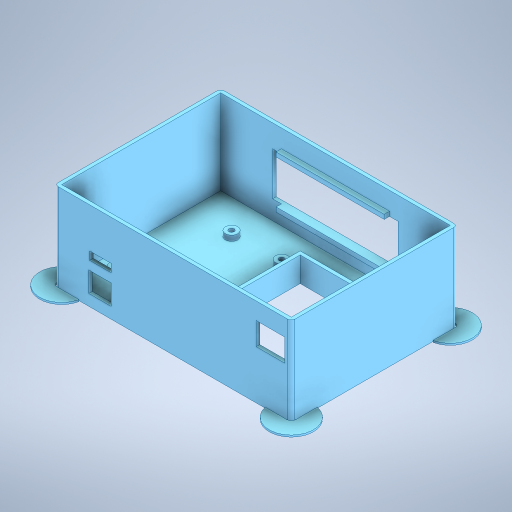
# Autodesk Inventor part: case_under_v2
Saved by Autodesk Inventor 2023 (Build 270158000, 158)
## iProperties
Created: 2022-09-15
Part Number: case_under_v2
Material: 일반
Document SubType Name: Modeling
Designer: 전상현
Density: 1 g/cm^3
Appearance: 기본값(1)
Author: 전상현
Autodesk Inventor part; units mm, degrees
ref_plane "YZ Plane" through (0, 0, 0) normal (1, 0, 0) x (0, 1, 0)
ref_plane "XZ Plane" through (0, 0, 0) normal (0, 1, 0) x (-1, 0, 0)
ref_plane "XY Plane" through (0, 0, 0) normal (0, 0, 1) x (1, 0, 0)
sketch "스케치1" plane through (0, 0, 0) normal (0, 1, 0) x (-1, 0, 0)
  line L0 (65, -45) -> (-65, -45)
  line L1 (-65, -45) -> (-65, 45)
  line L2 (-65, 45) -> (65, 45)
  line L3 (65, 45) -> (65, -45)
  line L4 (65, -45) -> (-65, 45) construction
  line L5 (-65, -45) -> (65, 45) construction
  line L6 (-67, -47) -> (67, -47)
  line L7 (67, -47) -> (67, 47)
  line L8 (67, 47) -> (-67, 47)
  line L9 (-67, 47) -> (-67, -47)
  line L10 (-1, -24) -> (-64, -24)
  line L11 (-64, -24) -> (-64, 34)
  line L12 (-64, 34) -> (-1, 34)
  line L13 (-1, 34) -> (-1, -24)
  circle A0 centre (-32.5, 39) radius 1.5
  circle A1 centre (-32.5, 39) radius 3.5
  arc A2 (-27.5, 39) -> (-37.5, 39) centre (-32.5, 39) ccw
  line L14 (-27.5, 39) -> (-27.5, 34)
  line L15 (-37.5, 39) -> (-37.5, 34)
  point P0 (0, 0)
  point P1 (-32.5, 34)
  point P2 (-32.5, 44)
  dimension "d0" = 130
  dimension "d1" = 90
  dimension "d2" = 2
  dimension "d3" = 58
  dimension "d4" = 63
  dimension "d5" = 3
  dimension "d6" = 7
  dimension "d7" = 10
  dimension "d8" = 1
  dimension "d9" = 1
  constraints: 32 end point, 6 parallel, 5 perpendicular, 4 midpoint, 3 centre point, 3 point on circle, 2 coincident, 2 horizontal, 2 point on line, 2 tangent, 2 vertical alignment, 3 other
  measures "d0" distance of L1.end L2.end
  measures "d1" distance of L0.end L1.end
  measures "d2" distance between parallel lines of L0 L6
  measures "d3" distance of L10.end L11.end
  measures "d4" distance of L10.start L10.end
  measures "d5" diameter of A0
  measures "d6" diameter of A1
  measures "d7" diameter of A2
  measures "d8" distance from line of L2 point (-32.5, 44)
  measures "d9" distance between parallel lines of L1 L11
extrude "돌출1" add sketch "스케치1" along normal blind 2 contours L0 L1 L2 L3 | L9 L8 L7 L6
extrude "돌출2" add sketch "스케치1" along normal blind 3 from surface at 2 contours L12 L15 A2 L14 | A1
sketch "스케치2" plane through (0, 2, 0) normal (0, 1, 0) x (1, 0, 0)
  line L0 (-67, -47) -> (67, -47) projected
  line L1 (67, -47) -> (67, 47) projected
  line L2 (67, 47) -> (-67, 47) projected
  line L3 (-67, 47) -> (-67, -47) projected
  line L4 (64, -34) -> (37.5, -34) projected
  line L5 (37.5, -34) -> (37.5, -39) projected
  arc A0 (27.5, -39) -> (37.5, -39) centre (32.5, -39) ccw projected
  line L6 (27.5, -39) -> (27.5, -34) projected
  line L7 (27.5, -34) -> (1, -34) projected
  line L8 (1, -34) -> (1, 24) projected
  line L9 (1, 24) -> (64, 24) projected
  line L10 (64, 24) -> (64, -34) projected
  line L11 (39, -39) -> (39, -35.5)
  line L12 (64, -55.5) -> (65.5, -55.5)
  line L13 (65.5, -55.5) -> (65.5, 25.5)
  line L14 (65.5, 25.5) -> (-0.5, 25.5)
  line L15 (-0.5, 25.5) -> (-0.5, -55.5)
  line L16 (-0.5, -55.5) -> (1, -55.5)
  line L17 (26, -55.5) -> (26, -39)
  arc A1 (26, -39) -> (39, -39) centre (32.5, -39) ccw
  line L18 (39, -35.5) -> (39, -34)
  line L19 (26, -55.5) -> (26, -34)
  point P0 (0, 0)
  dimension "d14" = 1.5
  constraints: 18 end point, 4 point on line, 2 point on circle, 1 centre point, 1 collinear, 1 parallel, 1 tangent, 1 vertical, 3 other
  measures "d14" radial gap between concentric circles of A0 A1
extrude "돌출3" add sketch "스케치2" along normal blind 3 contours L19 L7 L6 A0 L5 L4 L18 L11 A1
fillet "모깎기1" radius 1 2 edges at (32.5, 2, 45.5) (39, 2, 36.5)
extrude "돌출4" add sketch "스케치1" along normal blind 50 contours L9 L8 L7 L6
sketch "스케치3" plane through (0, 2, 0) normal (0, 1, 0) x (1, 0, 0)
  point P0 (0, 0)
sketch "스케치4" plane through (0, 2, 0) normal (0, 1, 0) x (1, 0, 0)
  line L0 (37, -45) -> (65, -45) projected
  line L1 (65, -45) -> (65, 45) projected
  line L2 (65, 45) -> (-65, 45) projected
  line L3 (-65, 45) -> (-65, -45) projected
  line L4 (-65, -45) -> (28, -45) projected
  arc A0 (25, -39) -> (28, -45) centre (32.5, -39) ccw projected
  line L5 (25, -34) -> (1, -34) projected
  line L6 (1, -34) -> (1, 24) projected
  line L7 (1, 24) -> (64, 24) projected
  line L8 (64, 24) -> (64, -34) projected
  line L9 (64, -34) -> (40, -34) projected
  line L10 (40, -39) -> (40, -34) projected
  arc A1 (37, -45) -> (40, -39) centre (32.5, -39) ccw projected
  line L11 (73.9957, 33.9957) -> (-8.9957, 33.9957)
  line L12 (-8.9957, 33.9957) -> (-8.9957, -43.9957)
  line L13 (-8.9957, -43.9957) -> (25.1098, -43.9957)
  line L14 (49.9957, -39) -> (49.9957, -43.9957)
  line L15 (49.9957, -43.9957) -> (73.9957, -43.9957)
  line L16 (73.9957, -43.9957) -> (73.9957, 33.9957)
  line L17 (-1, 26) -> (74.9957, 26)
  line L18 (74.9957, 26) -> (74.9957, -36)
  line L19 (74.9957, -36) -> (-1, -36)
  line L20 (-1, -36) -> (-1, 26)
  line L21 (25.1098, -36) -> (49.9957, -36)
  line L22 (49.9957, -43.9957) -> (25.1098, -43.9957)
  line L23 (25, -34) -> (25, -39) projected
  line L24 (25, -34) -> (40, -34)
  line L25 (64, -34) -> (37.5, -34) projected
  line L26 (25.1098, -36) -> (40, -36)
  point P0 (0, 0)
  point P1 (40, -36)
  point P2 (25, -36)
  point P3 (73.9957, -36)
  point P4 (73.9957, 26)
  point P5 (65, -36)
  point P6 (65, 26)
  dimension "d20" = 2
  dimension "d21" = 2
  dimension "d22" = 2
  dimension "d23" = 1
  constraints: 28 end point, 5 point on line, 3 parallel, 2 horizontal, 1 collinear, 1 perpendicular, 4 other
  measures "d20" distance between parallel lines of L17 L7
  measures "d21" distance between parallel lines of L9 L19
  measures "d22" distance between parallel lines of L6 L20
  measures "d23" distance between parallel lines of L18 L16
extrude "돌출5" add sketch "스케치4" along normal blind 12 contours L19 L10 L9 L8 L7 L6 L5 L23 L20 L17 L1 | L19 L23 L24 L10
sketch "스케치5" plane through (74.9957, 2, -26) normal (0, 0, -1) x (-1, 0, 0)
  line L0 (37.4957, 2.5) -> (47.4957, 2.5)
  line L1 (47.4957, 2.5) -> (47.4957, 0)
  line L2 (47.4957, 0) -> (37.4957, 0)
  line L3 (37.4957, 0) -> (37.4957, 2.5)
  line L4 (9.9957, 0) -> (75.9957, 0) projected
  line L5 (0, 0) -> (0, 12) projected
  point P0 (74.9957, -2)
  point P1 (39.9957, 0)
  point P2 (42.4957, 2.5)
  point P3 (10.9957, 12)
  point P4 (7.9957, 0)
  dimension "d28" = 2.5
  dimension "d29" = 10
  dimension "d93" = 31.5
  constraints: 8 end point, 2 parallel, 1 horizontal, 1 midpoint, 1 perpendicular, 1 point on line
  measures "d28" distance of L0.end L1.end
  measures "d29" distance of L0.start L0.end
  measures "d93" horizontal distance of point (10.996, 12) point (42.496, 2.5)
extrude "돌출6" cut sketch "스케치5" against normal up to surface (2 mm away)
sketch "스케치6" plane through (0, 2, 0) normal (0, 1, 0) x (1, 0, 0)
  line L0 (-3.7, -40.4) -> (-57, -40.4)
  line L1 (-57, -40.4) -> (-57, 28.2)
  line L2 (-57, 28.2) -> (-3.7, 28.2)
  line L3 (-3.7, 28.2) -> (-3.7, -40.4)
  line L4 (-3.7, 25.7) -> (-51.0807, 25.7)
  line L5 (-51.0807, 25.7) -> (-51.0807, 28.2)
  line L6 (-51.0807, 28.2) -> (-3.7, 28.2)
  line L7 (-3.7, 28.2) -> (-3.7, 25.7)
  line L8 (-51.0807, 25.7) -> (-57, 25.7)
  circle A0 centre (-11.15, 25.7) radius 1.5
  circle A1 centre (-39.55, 25.7) radius 1.5
  circle A2 centre (-54.75, -24.8) radius 1.5
  circle A3 centre (-6.45, -26.7) radius 1.5
  line L9 (-35.4, -40.4) -> (-47.4, -40.4)
  line L10 (-47.4, -40.4) -> (-47.4, -47)
  line L11 (-47.4, -47) -> (-35.4, -47)
  line L12 (-35.4, -47) -> (-35.4, -40.4)
  line L13 (-67, -47) -> (67, -47) projected
  line L14 (-65, -45) -> (-65, 45) projected
  circle A4 centre (-54.75, -24.8) radius 3.5
  circle A5 centre (-6.45, -26.7) radius 3.5
  circle A6 centre (-11.15, 25.7) radius 3.5
  circle A7 centre (-39.55, 25.7) radius 3.5
  point P0 (0, 0)
  point P1 (-41.4, -47)
  point P2 (-54.0404, 25.7)
  dimension "d33" = 53.3
  dimension "d34" = 68.6
  dimension "d36" = 3
  dimension "d37" = 3
  dimension "d38" = 28.4
  dimension "d39" = 3
  dimension "d40" = 3
  dimension "d41" = 52.4
  dimension "d42" = 50.5
  dimension "d44" = 15.2
  dimension "d45" = 4.7
  dimension "d46" = 2.25
  dimension "d47" = 12
  dimension "d48" = 9.6
  dimension "d49" = 6.6
  dimension "d50" = 8
  dimension "d51" = 2.5
  dimension "d52" = 2
  dimension "d53" = 2
  dimension "d54" = 2
  dimension "d55" = 2
  constraints: 26 end point, 8 centre point, 7 point on line, 6 parallel, 4 horizontal, 3 perpendicular, 2 midpoint
  measures "d33" distance of L0.start L0.end
  measures "d34" distance of L0.end L1.end
  measures "d36" diameter of A0
  measures "d37" diameter of A1
  measures "d38" distance of A1.centre A0.centre
  measures "d39" diameter of A2
  measures "d40" diameter of A3
  measures "d41" distance from line of L4 A3.centre
  measures "d42" distance from line of L8 A2.centre
  measures "d44" horizontal distance of A1.centre A2.centre
  measures "d45" horizontal distance of A0.centre A3.centre
  measures "d46" distance from line of L1 A2.centre
  measures "d47" distance of L10.end L11.end
  measures "d48" distance between parallel lines of L1 L10
  measures "d49" distance of L9.end L10.end
  measures "d50" distance between parallel lines of L14 L1
  measures "d51" distance from line of L2 point (-54.04, 25.7)
  measures "d52" radial gap between concentric circles of A2 A4
  measures "d53" radial gap between concentric circles of A3 A5
  measures "d54" radial gap between concentric circles of A0 A6
  measures "d55" radial gap between concentric circles of A1 A7
extrude "돌출7" add sketch "스케치6" along normal blind 3 contours A5 L3 | L3 A5 | A4 L1 | L1 A4 | A6 L4 A0 | L4 A0 A6 L2 | L2 A6 | A7 L4 A1 | L4 A1 A7 L2 | L2 A7
sketch "스케치7" plane through (65, 50, 45) normal (0, 0, -1) x (-1, 0, 0)
  line L0 (100.4, -32.5) -> (112.4, -32.5)
  line L1 (112.4, -32.5) -> (112.4, -43.4)
  line L2 (112.4, -43.4) -> (100.4, -43.4)
  line L3 (100.4, -43.4) -> (100.4, -32.5)
  line L4 (130, -48) -> (130, 0) projected
  line L5 (130, -48) -> (37, -48) projected
  line L6 (112.7, -32.2) -> (100.1, -32.2)
  line L7 (100.1, -32.2) -> (100.1, -43.7)
  line L8 (100.1, -43.7) -> (112.7, -43.7)
  line L9 (112.7, -43.7) -> (112.7, -32.2)
  point P0 (65, -50)
  dimension "d58" = 10.9
  dimension "d59" = 12
  dimension "d60" = 17.6
  dimension "d61" = 4.6
  dimension "d62" = 0.3
  constraints: 16 end point, 4 parallel, 2 perpendicular, 1 horizontal, 3 other
  measures "d58" distance of L0.end L1.end
  measures "d59" distance of L0.start L0.end
  measures "d60" distance between parallel lines of L4 L1
  measures "d61" distance between parallel lines of L5 L2
  measures "d62" distance between parallel lines of L0 L6
extrude "돌출8" cut sketch "스케치7" against normal through all contours L0 L1 L2 L3 | L9 L8 L7 L6
sketch "스케치8" plane through (67, 0, -47) normal (0, 0, -1) x (-1, 0, 0)
  line L0 (31.4, 37.25) -> (102.6, 37.25)
  line L1 (102.6, 37.25) -> (102.6, 12.75)
  line L2 (102.6, 12.75) -> (31.4, 12.75)
  line L3 (31.4, 12.75) -> (31.4, 37.25)
  line L4 (31.4, 37.25) -> (102.6, 12.75) construction
  line L5 (102.6, 37.25) -> (31.4, 12.75) construction
  line L6 (27, 43) -> (107, 43)
  line L7 (107, 43) -> (107, 7)
  line L8 (107, 7) -> (27, 7)
  line L9 (27, 7) -> (27, 43)
  line L10 (27, 43) -> (107, 7) construction
  line L11 (107, 43) -> (27, 7) construction
  circle A0 centre (104.5, 40.5) radius 1.6
  circle A1 centre (104.5, 9.5) radius 1.6
  circle A2 centre (29.5, 9.5) radius 1.6
  circle A3 centre (29.5, 40.5) radius 1.6
  line L12 (134, 0) -> (134, 50) projected
  point P0 (67, 0)
  point P1 (67, 25)
  point P2 (134, 25)
  dimension "d65" = 71.2
  dimension "d66" = 24.5
  dimension "d67" = 36
  dimension "d68" = 80
  dimension "d69" = 3.2
  dimension "d70" = 2.5
  dimension "d71" = 3.2
  dimension "d72" = 3.2
  dimension "d73" = 3.2
  dimension "d74" = 2.5
  dimension "d75" = 31
  dimension "d76" = 75
  dimension "d77" = 2.5
  constraints: 24 end point, 5 midpoint, 4 centre point, 4 parallel, 3 vertical alignment, 2 horizontal, 2 horizontal alignment, 2 perpendicular
  measures "d65" distance of L1.end L2.end
  measures "d66" distance of L0.end L1.end
  measures "d67" distance of L6.end L7.end
  measures "d68" distance of L6.start L6.end
  measures "d69" diameter of A0
  measures "d70" distance from line of L7 A0.centre
  measures "d71" diameter of A1
  measures "d72" diameter of A2
  measures "d73" diameter of A3
  measures "d74" distance from line of L9 A3.centre
  measures "d75" distance of A2.centre A3.centre
  measures "d76" distance of A0.centre A3.centre
  measures "d77" distance from line of L6 A3.centre
extrude "돌출9" cut sketch "스케치8" against normal up to surface (2 mm away) contours L0 L1 L2 L3
sketch "스케치9" plane through (65, 50, 45) normal (0, 0, -1) x (-1, 0, 0)
  line L0 (2, -10) -> (17.5, -10)
  line L1 (17.5, -10) -> (17.5, -22)
  line L2 (17.5, -22) -> (2, -22)
  line L3 (2, -22) -> (2, -10)
  line L4 (0, -48) -> (0, 0) projected
  line L5 (0, 0) -> (130, 0) projected
  line L6 (17.9, -9.6) -> (1.6, -9.6)
  line L7 (1.6, -9.6) -> (1.6, -22.4)
  line L8 (1.6, -22.4) -> (17.9, -22.4)
  line L9 (17.9, -22.4) -> (17.9, -9.6)
  point P0 (65, -50)
  point P1 (17.5, -16)
  dimension "d80" = 12
  dimension "d81" = 15.5
  dimension "d82" = 2
  dimension "d88" = 16
  dimension "d89" = 0.4
  constraints: 16 end point, 4 parallel, 2 perpendicular, 1 horizontal, 1 midpoint, 3 other
  measures "d80" distance of L2.end L0.start
  measures "d81" distance of L0.start L0.end
  measures "d82" distance between parallel lines of L4 L3
  measures "d88" distance from line of point (17.5, -16) L5
  measures "d89" distance between parallel lines of L0 L6
extrude "돌출10" cut sketch "스케치9" against normal through all contours L0 L1 L2 L3 | L9 L8 L7 L6
sketch "스케치10" plane through (65, 2, 45) normal (-1, 0, 0) x (0, 0, 1)
  line L0 (-9, 38.4) -> (-7, 38.4)
  line L1 (-7, 38.4) -> (-7, 25.6)
  line L2 (-7, 25.6) -> (-9, 25.6)
  line L3 (-9, 25.6) -> (-9, 38.4)
  line L4 (2, -2) -> (2, 48) projected
  line L5 (0, 25.6) -> (0, 38.4) projected
  point P0 (-45, -2)
  point P1 (-8, 38.4)
  point P2 (-8, 25.6)
  dimension "d86" = 2
  dimension "d87" = 9
  constraints: 8 end point, 2 horizontal alignment, 2 midpoint, 2 parallel, 1 horizontal, 1 perpendicular
  measures "d86" distance of L1.end L2.end
  measures "d87" distance between parallel lines of L4 L1
extrude "돌출11" add sketch "스케치10" along normal blind 10
sketch "스케치11" plane through (-65, 2, -45) normal (0, 0, 1) x (1, 0, 0)
  line L0 (34.4, 35.25) -> (95.6, 35.25)
  line L1 (95.6, 35.25) -> (95.6, 37.75)
  line L2 (95.6, 37.75) -> (34.4, 37.75)
  line L3 (34.4, 37.75) -> (34.4, 35.25)
  line L4 (29.4, 35.25) -> (29.4, 10.75) projected
  line L5 (29.4, 10.75) -> (100.6, 10.75) projected
  line L6 (100.6, 10.75) -> (100.6, 35.25) projected
  line L7 (100.6, 35.25) -> (29.4, 35.25) projected
  line L8 (132, -2) -> (-2, -2) projected
  line L9 (-2, -2) -> (-2, 48) projected
  line L10 (132, 48) -> (-2, 48) projected
  line L11 (132, -2) -> (132, 48) projected
  line L12 (34.4, 10.75) -> (95.6, 10.75)
  line L13 (95.6, 10.75) -> (95.6, 8.25)
  line L14 (95.6, 8.25) -> (34.4, 8.25)
  line L15 (34.4, 8.25) -> (34.4, 10.75)
  point P0 (65, -2)
  dimension "d94" = 2.5
  dimension "d95" = 5
  dimension "d96" = 5
  dimension "d97" = 2.5
  constraints: 16 end point, 4 parallel, 2 horizontal, 2 perpendicular, 2 point on line, 2 vertical alignment
  measures "d94" distance of L0.end L1.end
  measures "d95" distance between parallel lines of L6 L1
  measures "d96" distance between parallel lines of L3 L4
  measures "d97" distance of L12.end L13.end
extrude "돌출12" add sketch "스케치11" along normal blind 3 contours L3 L2 L1 L0 | L5 L13 L14 L15
fillet "모깎기2" radius 2 4 edges at (67, 25, -47) (-67, 25, -47) (-67, 25, 47) (67, 25, 47)
sketch "스케치12" plane through (0, 0, 0) normal (0, -1, 0) x (1, 0, 0)
  arc A0 (67, 45) -> (65, 47) centre (65, 45) ccw projected
  circle A1 centre (65, 45) radius 12.5
  arc A2 (67, 45) -> (65, 47) centre (65, 45) ccw projected
  line L0 (-65, 47) -> (65, 47) projected
  arc A3 (-65, 47) -> (-67, 45) centre (-65, 45) ccw projected
  line L1 (-67, -45) -> (-67, 45) projected
  arc A4 (-67, -45) -> (-65, -47) centre (-65, -45) ccw projected
  line L2 (65, -47) -> (-65, -47) projected
  arc A5 (65, -47) -> (67, -45) centre (65, -45) ccw projected
  line L3 (67, 45) -> (67, -45) projected
  line L4 (64, -24) -> (64, 34) projected
  line L5 (1, -24) -> (64, -24) projected
  line L6 (1, 34) -> (1, -24) projected
  line L7 (27.5, 34) -> (1, 34) projected
  line L8 (27.5, 39) -> (27.5, 34) projected
  arc A6 (37.5, 39) -> (27.5, 39) centre (32.5, 39) ccw projected
  line L9 (37.5, 34) -> (37.5, 39) projected
  line L10 (64, 34) -> (37.5, 34) projected
  line L11 (-65, 45) -> (28, 45) projected
  circle A7 centre (-65, 45) radius 12.5
  line L12 (-65, -45) -> (-65, 45) projected
  circle A8 centre (-65, -45) radius 12.5
  line L13 (65, 45) -> (65, -45) projected
  circle A9 centre (65, -45) radius 12.5
  arc A10 (-67.5, -45) -> (-65, -47.5) centre (-65, -45) ccw
  line L14 (-67.5, -45) -> (-67.5, 45)
  arc A11 (-65, 47.5) -> (-67.5, 45) centre (-65, 45) ccw
  line L15 (-65, 47.5) -> (65, 47.5)
  arc A12 (67.5, 45) -> (65, 47.5) centre (65, 45) ccw
  line L16 (67.5, 45) -> (67.5, -45)
  arc A13 (65, -47.5) -> (67.5, -45) centre (65, -45) ccw
  line L17 (65, -47.5) -> (-65, -47.5)
  point P0 (0, 0)
  point P1 (52.661, -47)
  point P2 (67, -32.661)
  point P3 (-67, -32.661)
  point P4 (-52.661, -47)
  point P5 (-52.661, 47)
  point P6 (-67, 32.661)
  point P7 (67, 32.661)
  point P8 (52.661, 47)
  point P9 (65, 47)
  point P10 (67.5, 32.7526)
  point P11 (52.7526, 47.5)
  point P12 (-52.7526, 47.5)
  point P13 (-67.5, 32.7526)
  point P14 (52.7526, -47.5)
  point P15 (67.5, -32.7526)
  point P16 (-67.5, -32.7526)
  point P17 (-52.7526, -47.5)
  dimension "d101" = 25
  dimension "d102" = 25
  dimension "d103" = 25
  dimension "d104" = 25
  dimension "d122" = 0.5
  constraints: 8 centre point, 8 end point, 8 point on circle, 4 coincident, 7 other
  measures "d101" diameter of A1
  measures "d102" diameter of A7
  measures "d103" diameter of A8
  measures "d104" diameter of A9
  measures "d122" distance between parallel lines of L2 L17
extrude "돌출13" add sketch "스케치12" against normal blind 1 contours L16 A12 L15 A1 | A9 L17 A13 L16 | L15 A11 L14 A7 | L14 A10 L17 A8
sketch "스케치15" plane through (-65, 50, 47) normal (0, 0, 1) x (1, 0, 0)
  line L0 (18.1, -22.9) -> (29.6, -22.9)
  line L1 (29.6, -22.9) -> (29.6, -26.9)
  line L2 (29.6, -26.9) -> (18.1, -26.9)
  line L3 (18.1, -26.9) -> (18.1, -22.9)
  line L4 (29.9, -22.6) -> (17.8, -22.6)
  line L5 (17.8, -22.6) -> (17.8, -27.2)
  line L6 (17.8, -27.2) -> (29.9, -27.2)
  line L7 (29.9, -27.2) -> (29.9, -22.6)
  line L8 (17.3, -32.2) -> (29.9, -32.2) projected
  point P0 (65, -50)
  point P1 (23.6, -32.2)
  point P2 (23.85, -27.2)
  dimension "d116" = 11.5
  dimension "d117" = 4
  dimension "d118" = 0.3
  dimension "d119" = 5
  constraints: 16 end point, 4 parallel, 2 midpoint, 2 perpendicular, 1 horizontal, 1 vertical alignment, 3 other
  measures "d116" distance of L1.end L2.end
  measures "d117" distance of L2.end L0.start
  measures "d118" distance between parallel lines of L0 L4
  measures "d119" vertical distance of point (23.6, -32.2) point (23.85, -27.2)
extrude "돌출14" cut sketch "스케치15" against normal blind 40 contours L0 L1 L2 L3 | L7 L6 L5 L4
